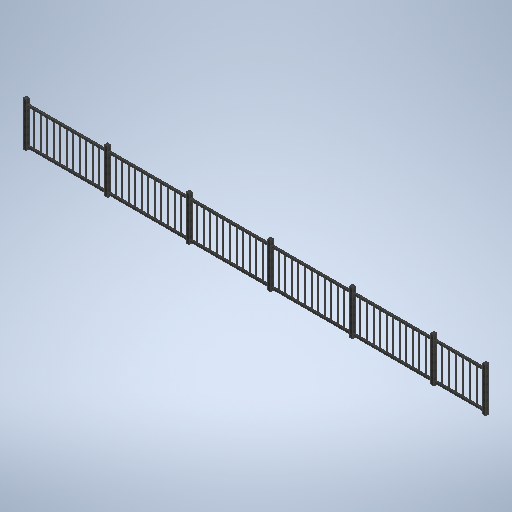
# Autodesk Inventor part: Railing side A
Saved by Autodesk Inventor 2025 (Build 290162000, 162)
## iProperties
Created: 2024-07-15
Part Number: Railing side A
Material: Steel ASTM A36
Document SubType Name: Modeling
Designer: track
Density: 7.85 g/cm^3
Appearance: Plate
Author: track
Autodesk Inventor part; units mm, degrees
ref_plane "YZ Plane" through (0, 0, 0) normal (1, 0, 0) x (0, 1, 0)
ref_plane "XZ Plane" through (0, 0, 0) normal (0, 1, 0) x (-1, 0, 0)
ref_plane "XY Plane" through (0, 0, 0) normal (0, 0, 1) x (1, 0, 0)
sketch "Sketch1" plane through (0, 0, 0) normal (0, 1, 0) x (-1, 0, 0)
  line L0 (-38.1, -38.1) -> (38.1, -38.1)
  line L1 (38.1, -38.1) -> (38.1, 38.1)
  line L2 (38.1, 38.1) -> (-38.1, 38.1)
  line L3 (-38.1, 38.1) -> (-38.1, -38.1)
  line L4 (-38.1, -38.1) -> (38.1, 38.1) construction
  line L5 (38.1, -38.1) -> (-38.1, 38.1) construction
  point P0 (0, 0)
  dimension "d0" = 76.2
  dimension "d1" = 76.2
  constraints: 12 end point, 2 midpoint, 2 parallel, 1 horizontal, 1 perpendicular
  measures "d0" distance of L1.end L2.end
  measures "d1" distance of L0.end L1.end
extrude "Extrusion1" add sketch "Sketch1" along normal blind 1117.6
sketch "Sketch2" plane through (38.1, 0, 38.1) normal (1, 0, 0) x (0, 0, -1)
  line L0 (19.05, 95.25) -> (57.15, 95.25)
  line L1 (57.15, 95.25) -> (57.15, 57.15)
  line L2 (57.15, 57.15) -> (19.05, 57.15)
  line L3 (19.05, 57.15) -> (19.05, 95.25)
  line L4 (19.05, 95.25) -> (57.15, 57.15) construction
  line L5 (57.15, 95.25) -> (19.05, 57.15) construction
  line L6 (19.05, 996.95) -> (57.15, 996.95)
  line L7 (57.15, 996.95) -> (57.15, 958.85)
  line L8 (57.15, 958.85) -> (19.05, 958.85)
  line L9 (19.05, 958.85) -> (19.05, 996.95)
  line L10 (19.05, 996.95) -> (57.15, 958.85) construction
  line L11 (57.15, 996.95) -> (19.05, 958.85) construction
  line L12 (76.2, 329.1929) -> (76.2, 1461.8329)
  line L13 (76.2, 282.1305) -> (76.2, 1152.2607)
  line L14 (76.2, 0) -> (76.2, 1117.6) projected
  line L15 (0, 0) -> (76.2, 0) projected
  point P0 (38.1, 0)
  point P1 (-393.2293, 273.1932)
  point P2 (483.6892, 252.9929)
  point P3 (38.1, 76.2)
  point P4 (38.1, 977.9)
  dimension "d4" = 38.1
  dimension "d5" = 38.1
  dimension "d6" = 38.1
  dimension "d7" = 863.6
  dimension "d8" = 38.1
  dimension "d9" = 38.1
  dimension "d10" = 38.1
  dimension "d12" = 76.2
  constraints: 28 end point, 4 midpoint, 4 parallel, 2 horizontal, 2 perpendicular, 1 collinear, 1 point on line, 1 vertical
  measures "d4" distance of L0.end L1.end
  measures "d5" distance of L0.start L0.end
  measures "d6" distance from line of L12 point (38.1, 76.2)
  measures "d7" distance between parallel lines of L8 L0
  measures "d8" distance of L6.end L7.end
  measures "d9" distance of L6.start L6.end
  measures "d10" distance from line of L13 point (38.1, 977.9)
  measures "d12" distance from line of L15 point (38.1, 76.2)
extrude "Extrusion2" add sketch "Sketch2" along normal blind 1974.85
sketch "Sketch3" plane through (0, 0, 0) normal (0, 1, 0) x (-1, 0, 0)
  line L0 (0, 0) -> (-2051.05, 0)
  line L1 (-38.1, -19.05) -> (-2012.95, -19.05) projected
  line L2 (-2012.95, 38.1) -> (-2089.15, 38.1)
  line L3 (-2089.15, 38.1) -> (-2089.15, -38.1)
  line L4 (-2089.15, -38.1) -> (-2012.95, -38.1)
  line L5 (-2012.95, -38.1) -> (-2012.95, 38.1)
  line L6 (-2012.95, 38.1) -> (-2089.15, -38.1) construction
  line L7 (-2089.15, 38.1) -> (-2012.95, -38.1) construction
  line L8 (-2012.95, -19.05) -> (-2012.95, 19.05) projected
  dimension "d15" = 76.2
  dimension "d16" = 76.2
  constraints: 14 end point, 3 parallel, 2 midpoint, 1 collinear, 1 horizontal, 1 perpendicular
  measures "d15" distance of L3.end L4.end
  measures "d16" distance of L2.end L3.end
extrude "Extrusion3" add sketch "Sketch3" along normal blind 1117.6
sketch "Sketch4" plane through (2089.15, 0, 38.1) normal (1, 0, 0) x (0, 0, -1)
  line L0 (57.15, 996.95) -> (57.15, 958.85) projected
  line L1 (57.15, 958.85) -> (57.15, 996.95) projected
  line L2 (19.05, 996.95) -> (57.15, 996.95) projected
  line L3 (57.15, 996.95) -> (19.05, 996.95) projected
  line L4 (19.05, 958.85) -> (19.05, 996.95) projected
  line L5 (19.05, 996.95) -> (19.05, 958.85) projected
  line L6 (57.15, 958.85) -> (19.05, 958.85) projected
  line L7 (19.05, 958.85) -> (57.15, 958.85) projected
  line L8 (57.15, 57.15) -> (19.05, 57.15) projected
  line L9 (19.05, 57.15) -> (57.15, 57.15) projected
  line L10 (19.05, 57.15) -> (19.05, 95.25) projected
  line L11 (19.05, 95.25) -> (19.05, 57.15) projected
  line L12 (19.05, 95.25) -> (57.15, 95.25) projected
  line L13 (57.15, 95.25) -> (19.05, 95.25) projected
  line L14 (57.15, 95.25) -> (57.15, 57.15) projected
  line L15 (57.15, 57.15) -> (57.15, 95.25) projected
  line L16 (19.05, 95.25) -> (57.15, 95.25)
  line L17 (57.15, 95.25) -> (57.15, 57.15)
  line L18 (57.15, 57.15) -> (19.05, 57.15)
  line L19 (19.05, 57.15) -> (19.05, 95.25)
  line L20 (19.05, 996.95) -> (57.15, 996.95)
  line L21 (57.15, 996.95) -> (57.15, 958.85)
  line L22 (57.15, 958.85) -> (19.05, 958.85)
  line L23 (19.05, 958.85) -> (19.05, 996.95)
  point P0 (38.1, 0)
  point P1 (19.05, 958.85)
  point P2 (19.05, 996.95)
  point P3 (19.05, 95.25)
  point P4 (19.05, 57.15)
  constraints: 16 end point, 4 parallel, 2 horizontal, 2 perpendicular
extrude "Extrusion4" add sketch "Sketch4" along normal blind 1984.375
sketch "Sketch5" plane through (0, 0, 0) normal (0, 1, 0) x (-1, 0, 0)
  line L0 (-4073.525, -19.05) -> (-4073.525, 19.05) projected
  line L1 (-4073.525, 0) -> (-4111.625, 0)
  line L2 (-4149.725, -38.1) -> (-4073.525, -38.1)
  line L3 (-4073.525, -38.1) -> (-4073.525, 38.1)
  line L4 (-4073.525, 38.1) -> (-4149.725, 38.1)
  line L5 (-4149.725, 38.1) -> (-4149.725, -38.1)
  line L6 (-4149.725, -38.1) -> (-4073.525, 38.1) construction
  line L7 (-4073.525, -38.1) -> (-4149.725, 38.1) construction
  line L8 (-4073.525, -19.05) -> (-4073.525, 19.05) projected
  point P0 (0, 0)
  dimension "d21" = 76.2
  dimension "d22" = 76.2
  constraints: 14 end point, 3 midpoint, 2 horizontal, 2 parallel, 1 collinear, 1 perpendicular
  measures "d21" distance of L2.start L2.end
  measures "d22" distance of L4.end L2.start
extrude "Extrusion5" add sketch "Sketch5" along normal blind 1117.6
sketch "Sketch6" plane through (4149.725, 0, 38.1) normal (1, 0, 0) x (0, 0, -1)
  line L0 (19.05, 95.25) -> (57.15, 95.25) projected
  line L1 (57.15, 95.25) -> (19.05, 95.25) projected
  line L2 (19.05, 57.15) -> (19.05, 95.25) projected
  line L3 (19.05, 95.25) -> (19.05, 57.15) projected
  line L4 (57.15, 95.25) -> (57.15, 57.15) projected
  line L5 (57.15, 57.15) -> (57.15, 95.25) projected
  line L6 (57.15, 57.15) -> (19.05, 57.15) projected
  line L7 (19.05, 57.15) -> (57.15, 57.15) projected
  line L8 (57.15, 996.95) -> (57.15, 958.85) projected
  line L9 (57.15, 958.85) -> (57.15, 996.95) projected
  line L10 (57.15, 958.85) -> (19.05, 958.85) projected
  line L11 (19.05, 958.85) -> (57.15, 958.85) projected
  line L12 (19.05, 996.95) -> (57.15, 996.95) projected
  line L13 (57.15, 996.95) -> (19.05, 996.95) projected
  line L14 (19.05, 958.85) -> (19.05, 996.95) projected
  line L15 (19.05, 996.95) -> (19.05, 958.85) projected
  point P0 (38.1, 0)
extrude "Extrusion6" add sketch "Sketch6" along normal blind 1984.375
sketch "Sketch7" plane through (0, 0, 0) normal (0, 1, 0) x (-1, 0, 0)
  line L0 (-6134.1, 19.05) -> (-6134.1, -19.05) projected
  line L1 (-6134.1, 0) -> (-6172.2, 0)
  line L2 (-6134.1, 38.1) -> (-6210.3, 38.1)
  line L3 (-6210.3, 38.1) -> (-6210.3, -38.1)
  line L4 (-6210.3, -38.1) -> (-6134.1, -38.1)
  line L5 (-6134.1, -38.1) -> (-6134.1, 38.1)
  line L6 (-6134.1, 38.1) -> (-6210.3, -38.1) construction
  line L7 (-6210.3, 38.1) -> (-6134.1, -38.1) construction
  line L8 (-6134.1, -19.05) -> (-6134.1, 19.05) projected
  point P0 (0, 0)
  dimension "d27" = 76.2
  dimension "d28" = 76.2
  constraints: 14 end point, 3 midpoint, 2 horizontal, 2 parallel, 1 collinear, 1 perpendicular
  measures "d27" distance of L4.end L2.start
  measures "d28" distance of L3.end L4.end
extrude "Extrusion7" add sketch "Sketch7" along normal blind 1117.6
sketch "Sketch8" plane through (6210.3, 0, 38.1) normal (1, 0, 0) x (0, 0, -1)
  line L0 (19.05, 958.85) -> (19.05, 996.95) projected
  line L1 (19.05, 996.95) -> (19.05, 958.85) projected
  line L2 (19.05, 996.95) -> (57.15, 996.95) projected
  line L3 (57.15, 996.95) -> (19.05, 996.95) projected
  line L4 (57.15, 996.95) -> (57.15, 958.85) projected
  line L5 (57.15, 958.85) -> (57.15, 996.95) projected
  line L6 (57.15, 958.85) -> (19.05, 958.85) projected
  line L7 (19.05, 958.85) -> (57.15, 958.85) projected
  line L8 (57.15, 95.25) -> (57.15, 57.15) projected
  line L9 (57.15, 57.15) -> (57.15, 95.25) projected
  line L10 (57.15, 57.15) -> (19.05, 57.15) projected
  line L11 (19.05, 57.15) -> (57.15, 57.15) projected
  line L12 (19.05, 95.25) -> (57.15, 95.25) projected
  line L13 (57.15, 95.25) -> (19.05, 95.25) projected
  line L14 (19.05, 57.15) -> (19.05, 95.25) projected
  line L15 (19.05, 95.25) -> (19.05, 57.15) projected
  point P0 (38.1, 0)
extrude "Extrusion8" add sketch "Sketch8" along normal blind 1984.375
sketch "Sketch9" plane through (0, 0, 0) normal (0, 1, 0) x (-1, 0, 0)
  line L0 (-8194.675, 19.05) -> (-8194.675, -19.05) projected
  line L1 (-8194.675, 0) -> (-8232.775, 0)
  line L2 (-8194.675, 38.1) -> (-8270.875, 38.1)
  line L3 (-8270.875, 38.1) -> (-8270.875, -38.1)
  line L4 (-8270.875, -38.1) -> (-8194.675, -38.1)
  line L5 (-8194.675, -38.1) -> (-8194.675, 38.1)
  line L6 (-8194.675, 38.1) -> (-8270.875, -38.1) construction
  line L7 (-8270.875, 38.1) -> (-8194.675, -38.1) construction
  line L8 (-8194.675, -19.05) -> (-8194.675, 19.05) projected
  point P0 (0, 0)
  dimension "d33" = 76.2
  dimension "d34" = 76.2
  constraints: 14 end point, 3 midpoint, 2 horizontal, 2 parallel, 1 collinear, 1 perpendicular
  measures "d33" distance of L3.end L4.end
  measures "d34" distance of L4.end L2.start
extrude "Extrusion9" add sketch "Sketch9" along normal blind 1117.6
sketch "Sketch10" plane through (8270.875, 0, 38.1) normal (1, 0, 0) x (0, 0, -1)
  line L0 (19.05, 57.15) -> (19.05, 95.25) projected
  line L1 (19.05, 95.25) -> (19.05, 57.15) projected
  line L2 (19.05, 95.25) -> (57.15, 95.25) projected
  line L3 (57.15, 95.25) -> (19.05, 95.25) projected
  line L4 (57.15, 95.25) -> (57.15, 57.15) projected
  line L5 (57.15, 57.15) -> (57.15, 95.25) projected
  line L6 (57.15, 57.15) -> (19.05, 57.15) projected
  line L7 (19.05, 57.15) -> (57.15, 57.15) projected
  line L8 (57.15, 958.85) -> (19.05, 958.85) projected
  line L9 (19.05, 958.85) -> (57.15, 958.85) projected
  line L10 (57.15, 996.95) -> (57.15, 958.85) projected
  line L11 (57.15, 958.85) -> (57.15, 996.95) projected
  line L12 (19.05, 996.95) -> (57.15, 996.95) projected
  line L13 (57.15, 996.95) -> (19.05, 996.95) projected
  line L14 (19.05, 958.85) -> (19.05, 996.95) projected
  line L15 (19.05, 996.95) -> (19.05, 958.85) projected
  point P0 (38.1, 0)
extrude "Extrusion10" add sketch "Sketch10" along normal blind 1981.2
sketch "Sketch11" plane through (0, 0, 0) normal (0, 1, 0) x (-1, 0, 0)
  line L0 (-10252.075, 19.05) -> (-10252.075, -19.05) projected
  line L1 (-10252.075, 0) -> (-10290.175, 0)
  line L2 (-10328.275, 38.1) -> (-10252.075, 38.1)
  line L3 (-10252.075, 38.1) -> (-10252.075, -38.1)
  line L4 (-10252.075, -38.1) -> (-10328.275, -38.1)
  line L5 (-10328.275, -38.1) -> (-10328.275, 38.1)
  line L6 (-10328.275, 38.1) -> (-10252.075, -38.1) construction
  line L7 (-10252.075, 38.1) -> (-10328.275, -38.1) construction
  line L8 (-10252.075, -19.05) -> (-10252.075, 19.05) projected
  point P0 (0, 0)
  dimension "d39" = 76.2
  dimension "d40" = 76.2
  constraints: 14 end point, 3 midpoint, 2 horizontal, 2 parallel, 1 collinear, 1 perpendicular
  measures "d39" distance of L4.end L2.start
  measures "d40" distance of L3.end L4.end
extrude "Extrusion11" add sketch "Sketch11" along normal blind 1117.6
sketch "Sketch12" plane through (10328.275, 0, 38.1) normal (1, 0, 0) x (0, 0, -1)
  line L0 (19.05, 57.15) -> (19.05, 95.25) projected
  line L1 (19.05, 95.25) -> (19.05, 57.15) projected
  line L2 (19.05, 95.25) -> (57.15, 95.25) projected
  line L3 (57.15, 95.25) -> (19.05, 95.25) projected
  line L4 (57.15, 95.25) -> (57.15, 57.15) projected
  line L5 (57.15, 57.15) -> (57.15, 95.25) projected
  line L6 (57.15, 57.15) -> (19.05, 57.15) projected
  line L7 (19.05, 57.15) -> (57.15, 57.15) projected
  line L8 (57.15, 958.85) -> (19.05, 958.85) projected
  line L9 (19.05, 958.85) -> (57.15, 958.85) projected
  line L10 (57.15, 996.95) -> (57.15, 958.85) projected
  line L11 (57.15, 958.85) -> (57.15, 996.95) projected
  line L12 (19.05, 996.95) -> (57.15, 996.95) projected
  line L13 (57.15, 996.95) -> (19.05, 996.95) projected
  line L14 (19.05, 958.85) -> (19.05, 996.95) projected
  line L15 (19.05, 996.95) -> (19.05, 958.85) projected
  point P0 (38.1, 0)
  point P1 (76.2, 0)
extrude "Extrusion12" add sketch "Sketch12" along normal blind 1231.9
sketch "Sketch13" plane through (0, 0, 0) normal (0, 1, 0) x (-1, 0, 0)
  line L0 (-11560.175, 19.05) -> (-11560.175, -19.05) projected
  line L1 (-11560.175, 0) -> (-11598.275, 0)
  line L2 (-11560.175, 38.1) -> (-11636.375, 38.1)
  line L3 (-11636.375, 38.1) -> (-11636.375, -38.1)
  line L4 (-11636.375, -38.1) -> (-11560.175, -38.1)
  line L5 (-11560.175, -38.1) -> (-11560.175, 38.1)
  line L6 (-11560.175, 38.1) -> (-11636.375, -38.1) construction
  line L7 (-11636.375, 38.1) -> (-11560.175, -38.1) construction
  line L8 (-11560.175, -19.05) -> (-11560.175, 19.05) projected
  point P0 (0, 0)
  dimension "d45" = 76.2
  dimension "d46" = 76.2
  constraints: 14 end point, 3 midpoint, 2 horizontal, 2 parallel, 1 collinear, 1 perpendicular
  measures "d45" distance of L3.end L4.end
  measures "d46" distance of L2.end L3.end
extrude "Extrusion13" add sketch "Sketch13" along normal blind 1117.6
sketch "Sketch14" plane through (38.1, 95.25, 19.05) normal (0, 1, 0) x (1, 0, 0)
  line L0 (0, 0) -> (0, 38.1) projected
  line L1 (0, 19.05) -> (11598.275, 19.05) construction
  line L2 (11598.275, -19.05) -> (11598.275, 57.15) projected
  line L3 (158.2208, 12.7) -> (170.9208, 12.7)
  line L4 (170.9208, 12.7) -> (170.9208, 25.4)
  line L5 (170.9208, 25.4) -> (158.2208, 25.4)
  line L6 (158.2208, 25.4) -> (158.2208, 12.7)
  line L7 (158.2208, 12.7) -> (170.9208, 25.4) construction
  line L8 (170.9208, 12.7) -> (158.2208, 25.4) construction
  line L9 (322.7917, 12.7) -> (335.4917, 12.7)
  line L10 (335.4917, 12.7) -> (335.4917, 25.4)
  line L11 (335.4917, 25.4) -> (322.7917, 25.4)
  line L12 (322.7917, 25.4) -> (322.7917, 12.7)
  line L13 (487.3625, 12.7) -> (500.0625, 12.7)
  line L14 (500.0625, 12.7) -> (500.0625, 25.4)
  line L15 (500.0625, 25.4) -> (487.3625, 25.4)
  line L16 (487.3625, 25.4) -> (487.3625, 12.7)
  line L17 (651.9333, 12.7) -> (664.6333, 12.7)
  line L18 (664.6333, 12.7) -> (664.6333, 25.4)
  line L19 (664.6333, 25.4) -> (651.9333, 25.4)
  line L20 (651.9333, 25.4) -> (651.9333, 12.7)
  line L21 (816.5042, 12.7) -> (829.2042, 12.7)
  line L22 (829.2042, 12.7) -> (829.2042, 25.4)
  line L23 (829.2042, 25.4) -> (816.5042, 25.4)
  line L24 (816.5042, 25.4) -> (816.5042, 12.7)
  line L25 (981.075, 12.7) -> (993.775, 12.7)
  line L26 (993.775, 12.7) -> (993.775, 25.4)
  line L27 (993.775, 25.4) -> (981.075, 25.4)
  line L28 (981.075, 25.4) -> (981.075, 12.7)
  line L29 (1145.6458, 12.7) -> (1158.3458, 12.7)
  line L30 (1158.3458, 12.7) -> (1158.3458, 25.4)
  line L31 (1158.3458, 25.4) -> (1145.6458, 25.4)
  line L32 (1145.6458, 25.4) -> (1145.6458, 12.7)
  line L33 (1310.2167, 12.7) -> (1322.9167, 12.7)
  line L34 (1322.9167, 12.7) -> (1322.9167, 25.4)
  line L35 (1322.9167, 25.4) -> (1310.2167, 25.4)
  line L36 (1310.2167, 25.4) -> (1310.2167, 12.7)
  line L37 (1474.7875, 12.7) -> (1487.4875, 12.7)
  line L38 (1487.4875, 12.7) -> (1487.4875, 25.4)
  line L39 (1487.4875, 25.4) -> (1474.7875, 25.4)
  line L40 (1474.7875, 25.4) -> (1474.7875, 12.7)
  line L41 (1639.3583, 12.7) -> (1652.0583, 12.7)
  line L42 (1652.0583, 12.7) -> (1652.0583, 25.4)
  line L43 (1652.0583, 25.4) -> (1639.3583, 25.4)
  line L44 (1639.3583, 25.4) -> (1639.3583, 12.7)
  line L45 (1803.9292, 12.7) -> (1816.6292, 12.7)
  line L46 (1816.6292, 12.7) -> (1816.6292, 25.4)
  line L47 (1816.6292, 25.4) -> (1803.9292, 25.4)
  line L48 (1803.9292, 25.4) -> (1803.9292, 12.7)
  line L49 (2210.0646, 12.7) -> (2222.7646, 12.7)
  line L50 (2222.7646, 12.7) -> (2222.7646, 25.4)
  line L51 (2222.7646, 25.4) -> (2210.0646, 25.4)
  line L52 (2210.0646, 25.4) -> (2210.0646, 12.7)
  line L53 (2210.0646, 12.7) -> (2222.7646, 25.4) construction
  line L54 (2222.7646, 12.7) -> (2210.0646, 25.4) construction
  line L55 (2051.05, 0) -> (2051.05, 38.1) projected
  line L56 (2388.1292, 25.4) -> (2375.4292, 25.4)
  line L57 (2375.4292, 25.4) -> (2375.4292, 12.7)
  line L58 (2388.1292, 12.7) -> (2388.1292, 25.4)
  line L59 (2375.4292, 12.7) -> (2388.1292, 12.7)
  line L60 (2553.4938, 25.4) -> (2540.7938, 25.4)
  line L61 (2540.7938, 25.4) -> (2540.7938, 12.7)
  line L62 (2553.4938, 12.7) -> (2553.4938, 25.4)
  line L63 (2540.7938, 12.7) -> (2553.4938, 12.7)
  line L64 (2718.8583, 25.4) -> (2706.1583, 25.4)
  line L65 (2706.1583, 25.4) -> (2706.1583, 12.7)
  line L66 (2718.8583, 12.7) -> (2718.8583, 25.4)
  line L67 (2706.1583, 12.7) -> (2718.8583, 12.7)
  line L68 (2884.2229, 25.4) -> (2871.5229, 25.4)
  line L69 (2871.5229, 25.4) -> (2871.5229, 12.7)
  line L70 (2884.2229, 12.7) -> (2884.2229, 25.4)
  line L71 (2871.5229, 12.7) -> (2884.2229, 12.7)
  line L72 (3049.5875, 25.4) -> (3036.8875, 25.4)
  line L73 (3036.8875, 25.4) -> (3036.8875, 12.7)
  line L74 (3049.5875, 12.7) -> (3049.5875, 25.4)
  line L75 (3036.8875, 12.7) -> (3049.5875, 12.7)
  line L76 (3214.9521, 25.4) -> (3202.2521, 25.4)
  line L77 (3202.2521, 25.4) -> (3202.2521, 12.7)
  line L78 (3214.9521, 12.7) -> (3214.9521, 25.4)
  line L79 (3202.2521, 12.7) -> (3214.9521, 12.7)
  line L80 (3380.3167, 25.4) -> (3367.6167, 25.4)
  line L81 (3367.6167, 25.4) -> (3367.6167, 12.7)
  line L82 (3380.3167, 12.7) -> (3380.3167, 25.4)
  line L83 (3367.6167, 12.7) -> (3380.3167, 12.7)
  line L84 (3545.6813, 25.4) -> (3532.9813, 25.4)
  line L85 (3532.9813, 25.4) -> (3532.9813, 12.7)
  line L86 (3545.6813, 12.7) -> (3545.6813, 25.4)
  line L87 (3532.9813, 12.7) -> (3545.6813, 12.7)
  line L88 (3711.0458, 25.4) -> (3698.3458, 25.4)
  line L89 (3698.3458, 25.4) -> (3698.3458, 12.7)
  line L90 (3711.0458, 12.7) -> (3711.0458, 25.4)
  line L91 (3698.3458, 12.7) -> (3711.0458, 12.7)
  line L92 (3876.4104, 25.4) -> (3863.7104, 25.4)
  line L93 (3863.7104, 25.4) -> (3863.7104, 12.7)
  line L94 (3876.4104, 12.7) -> (3876.4104, 25.4)
  line L95 (3863.7104, 12.7) -> (3876.4104, 12.7)
  line L96 (4270.6396, 12.7) -> (4283.3396, 12.7)
  line L97 (4283.3396, 12.7) -> (4283.3396, 25.4)
  line L98 (4283.3396, 25.4) -> (4270.6396, 25.4)
  line L99 (4270.6396, 25.4) -> (4270.6396, 12.7)
  line L100 (4270.6396, 12.7) -> (4283.3396, 25.4) construction
  line L101 (4283.3396, 12.7) -> (4270.6396, 25.4) construction
  line L102 (4111.625, 0) -> (4111.625, 38.1) projected
  line L103 (4448.7042, 12.7) -> (4448.7042, 25.4)
  line L104 (4448.7042, 25.4) -> (4436.0042, 25.4)
  line L105 (4436.0042, 25.4) -> (4436.0042, 12.7)
  line L106 (4436.0042, 12.7) -> (4448.7042, 12.7)
  line L107 (4614.0688, 12.7) -> (4614.0688, 25.4)
  line L108 (4614.0688, 25.4) -> (4601.3688, 25.4)
  line L109 (4601.3688, 25.4) -> (4601.3688, 12.7)
  line L110 (4601.3688, 12.7) -> (4614.0688, 12.7)
  line L111 (4779.4333, 12.7) -> (4779.4333, 25.4)
  line L112 (4779.4333, 25.4) -> (4766.7333, 25.4)
  line L113 (4766.7333, 25.4) -> (4766.7333, 12.7)
  line L114 (4766.7333, 12.7) -> (4779.4333, 12.7)
  line L115 (4944.7979, 12.7) -> (4944.7979, 25.4)
  line L116 (4944.7979, 25.4) -> (4932.0979, 25.4)
  line L117 (4932.0979, 25.4) -> (4932.0979, 12.7)
  line L118 (4932.0979, 12.7) -> (4944.7979, 12.7)
  line L119 (5110.1625, 12.7) -> (5110.1625, 25.4)
  line L120 (5110.1625, 25.4) -> (5097.4625, 25.4)
  line L121 (5097.4625, 25.4) -> (5097.4625, 12.7)
  line L122 (5097.4625, 12.7) -> (5110.1625, 12.7)
  line L123 (5275.5271, 12.7) -> (5275.5271, 25.4)
  line L124 (5275.5271, 25.4) -> (5262.8271, 25.4)
  line L125 (5262.8271, 25.4) -> (5262.8271, 12.7)
  line L126 (5262.8271, 12.7) -> (5275.5271, 12.7)
  line L127 (5440.8917, 12.7) -> (5440.8917, 25.4)
  line L128 (5440.8917, 25.4) -> (5428.1917, 25.4)
  line L129 (5428.1917, 25.4) -> (5428.1917, 12.7)
  line L130 (5428.1917, 12.7) -> (5440.8917, 12.7)
  line L131 (5606.2563, 12.7) -> (5606.2563, 25.4)
  line L132 (5606.2563, 25.4) -> (5593.5563, 25.4)
  line L133 (5593.5563, 25.4) -> (5593.5563, 12.7)
  line L134 (5593.5563, 12.7) -> (5606.2563, 12.7)
  line L135 (5771.6208, 12.7) -> (5771.6208, 25.4)
  line L136 (5771.6208, 25.4) -> (5758.9208, 25.4)
  line L137 (5758.9208, 25.4) -> (5758.9208, 12.7)
  line L138 (5758.9208, 12.7) -> (5771.6208, 12.7)
  line L139 (5936.9854, 12.7) -> (5936.9854, 25.4)
  line L140 (5936.9854, 25.4) -> (5924.2854, 25.4)
  line L141 (5924.2854, 25.4) -> (5924.2854, 12.7)
  line L142 (5924.2854, 12.7) -> (5936.9854, 12.7)
  line L143 (6331.2146, 12.7) -> (6343.9146, 12.7)
  line L144 (6343.9146, 12.7) -> (6343.9146, 25.4)
  line L145 (6343.9146, 25.4) -> (6331.2146, 25.4)
  line L146 (6331.2146, 25.4) -> (6331.2146, 12.7)
  line L147 (6331.2146, 12.7) -> (6343.9146, 25.4) construction
  line L148 (6343.9146, 12.7) -> (6331.2146, 25.4) construction
  line L149 (6172.2, 0) -> (6172.2, 38.1) projected
  line L150 (6509.2792, 25.4) -> (6496.5792, 25.4)
  line L151 (6509.2792, 12.7) -> (6509.2792, 25.4)
  line L152 (6496.5792, 25.4) -> (6496.5792, 12.7)
  line L153 (6496.5792, 12.7) -> (6509.2792, 12.7)
  line L154 (6674.6438, 25.4) -> (6661.9438, 25.4)
  line L155 (6674.6438, 12.7) -> (6674.6438, 25.4)
  line L156 (6661.9438, 25.4) -> (6661.9438, 12.7)
  line L157 (6661.9438, 12.7) -> (6674.6438, 12.7)
  line L158 (6840.0083, 25.4) -> (6827.3083, 25.4)
  line L159 (6840.0083, 12.7) -> (6840.0083, 25.4)
  line L160 (6827.3083, 25.4) -> (6827.3083, 12.7)
  line L161 (6827.3083, 12.7) -> (6840.0083, 12.7)
  line L162 (7005.3729, 25.4) -> (6992.6729, 25.4)
  line L163 (7005.3729, 12.7) -> (7005.3729, 25.4)
  line L164 (6992.6729, 25.4) -> (6992.6729, 12.7)
  line L165 (6992.6729, 12.7) -> (7005.3729, 12.7)
  line L166 (7170.7375, 25.4) -> (7158.0375, 25.4)
  line L167 (7170.7375, 12.7) -> (7170.7375, 25.4)
  line L168 (7158.0375, 25.4) -> (7158.0375, 12.7)
  line L169 (7158.0375, 12.7) -> (7170.7375, 12.7)
  line L170 (7336.1021, 25.4) -> (7323.4021, 25.4)
  line L171 (7336.1021, 12.7) -> (7336.1021, 25.4)
  line L172 (7323.4021, 25.4) -> (7323.4021, 12.7)
  line L173 (7323.4021, 12.7) -> (7336.1021, 12.7)
  line L174 (7501.4667, 25.4) -> (7488.7667, 25.4)
  line L175 (7501.4667, 12.7) -> (7501.4667, 25.4)
  line L176 (7488.7667, 25.4) -> (7488.7667, 12.7)
  line L177 (7488.7667, 12.7) -> (7501.4667, 12.7)
  line L178 (7666.8313, 25.4) -> (7654.1313, 25.4)
  line L179 (7666.8313, 12.7) -> (7666.8313, 25.4)
  line L180 (7654.1313, 25.4) -> (7654.1313, 12.7)
  line L181 (7654.1313, 12.7) -> (7666.8313, 12.7)
  line L182 (7832.1958, 25.4) -> (7819.4958, 25.4)
  line L183 (7832.1958, 12.7) -> (7832.1958, 25.4)
  line L184 (7819.4958, 25.4) -> (7819.4958, 12.7)
  line L185 (7819.4958, 12.7) -> (7832.1958, 12.7)
  line L186 (7997.5604, 25.4) -> (7984.8604, 25.4)
  line L187 (7997.5604, 12.7) -> (7997.5604, 25.4)
  line L188 (7984.8604, 25.4) -> (7984.8604, 12.7)
  line L189 (7984.8604, 12.7) -> (7997.5604, 12.7)
  line L190 (8391.525, 12.7) -> (8404.225, 12.7)
  line L191 (8404.225, 12.7) -> (8404.225, 25.4)
  line L192 (8404.225, 25.4) -> (8391.525, 25.4)
  line L193 (8391.525, 25.4) -> (8391.525, 12.7)
  line L194 (8391.525, 12.7) -> (8404.225, 25.4) construction
  line L195 (8404.225, 12.7) -> (8391.525, 25.4) construction
  line L196 (8232.775, 0) -> (8232.775, 38.1) projected
  line L197 (8569.325, 12.7) -> (8569.325, 25.4)
  line L198 (8569.325, 25.4) -> (8556.625, 25.4)
  line L199 (8556.625, 25.4) -> (8556.625, 12.7)
  line L200 (8556.625, 12.7) -> (8569.325, 12.7)
  line L201 (8734.425, 12.7) -> (8734.425, 25.4)
  line L202 (8734.425, 25.4) -> (8721.725, 25.4)
  line L203 (8721.725, 25.4) -> (8721.725, 12.7)
  line L204 (8721.725, 12.7) -> (8734.425, 12.7)
  line L205 (8899.525, 12.7) -> (8899.525, 25.4)
  line L206 (8899.525, 25.4) -> (8886.825, 25.4)
  line L207 (8886.825, 25.4) -> (8886.825, 12.7)
  line L208 (8886.825, 12.7) -> (8899.525, 12.7)
  line L209 (9064.625, 12.7) -> (9064.625, 25.4)
  line L210 (9064.625, 25.4) -> (9051.925, 25.4)
  line L211 (9051.925, 25.4) -> (9051.925, 12.7)
  line L212 (9051.925, 12.7) -> (9064.625, 12.7)
  line L213 (9229.725, 12.7) -> (9229.725, 25.4)
  line L214 (9229.725, 25.4) -> (9217.025, 25.4)
  line L215 (9217.025, 25.4) -> (9217.025, 12.7)
  line L216 (9217.025, 12.7) -> (9229.725, 12.7)
  line L217 (9394.825, 12.7) -> (9394.825, 25.4)
  line L218 (9394.825, 25.4) -> (9382.125, 25.4)
  line L219 (9382.125, 25.4) -> (9382.125, 12.7)
  line L220 (9382.125, 12.7) -> (9394.825, 12.7)
  line L221 (9559.925, 12.7) -> (9559.925, 25.4)
  line L222 (9559.925, 25.4) -> (9547.225, 25.4)
  line L223 (9547.225, 25.4) -> (9547.225, 12.7)
  line L224 (9547.225, 12.7) -> (9559.925, 12.7)
  line L225 (9725.025, 12.7) -> (9725.025, 25.4)
  line L226 (9725.025, 25.4) -> (9712.325, 25.4)
  line L227 (9712.325, 25.4) -> (9712.325, 12.7)
  line L228 (9712.325, 12.7) -> (9725.025, 12.7)
  line L229 (9890.125, 12.7) -> (9890.125, 25.4)
  line L230 (9890.125, 25.4) -> (9877.425, 25.4)
  line L231 (9877.425, 25.4) -> (9877.425, 12.7)
  line L232 (9877.425, 12.7) -> (9890.125, 12.7)
  line L233 (10055.225, 12.7) -> (10055.225, 25.4)
  line L234 (10055.225, 25.4) -> (10042.525, 25.4)
  line L235 (10042.525, 25.4) -> (10042.525, 12.7)
  line L236 (10042.525, 12.7) -> (10055.225, 12.7)
  line L237 (10459.8107, 12.7) -> (10472.5107, 12.7)
  line L238 (10472.5107, 12.7) -> (10472.5107, 25.4)
  line L239 (10472.5107, 25.4) -> (10459.8107, 25.4)
  line L240 (10459.8107, 25.4) -> (10459.8107, 12.7)
  line L241 (10459.8107, 12.7) -> (10472.5107, 25.4) construction
  line L242 (10472.5107, 12.7) -> (10459.8107, 25.4) construction
  line L243 (10290.175, 0) -> (10290.175, 38.1) projected
  line L244 (10648.4964, 12.7) -> (10648.4964, 25.4)
  line L245 (10648.4964, 25.4) -> (10635.7964, 25.4)
  line L246 (10635.7964, 25.4) -> (10635.7964, 12.7)
  line L247 (10635.7964, 12.7) -> (10648.4964, 12.7)
  line L248 (10824.4821, 12.7) -> (10824.4821, 25.4)
  line L249 (10824.4821, 25.4) -> (10811.7821, 25.4)
  line L250 (10811.7821, 25.4) -> (10811.7821, 12.7)
  line L251 (10811.7821, 12.7) -> (10824.4821, 12.7)
  line L252 (11000.4679, 12.7) -> (11000.4679, 25.4)
  line L253 (11000.4679, 25.4) -> (10987.7679, 25.4)
  line L254 (10987.7679, 25.4) -> (10987.7679, 12.7)
  line L255 (10987.7679, 12.7) -> (11000.4679, 12.7)
  line L256 (11176.4536, 12.7) -> (11176.4536, 25.4)
  line L257 (11176.4536, 25.4) -> (11163.7536, 25.4)
  line L258 (11163.7536, 25.4) -> (11163.7536, 12.7)
  line L259 (11163.7536, 12.7) -> (11176.4536, 12.7)
  line L260 (11352.4393, 12.7) -> (11352.4393, 25.4)
  line L261 (11352.4393, 25.4) -> (11339.7393, 25.4)
  line L262 (11339.7393, 25.4) -> (11339.7393, 12.7)
  line L263 (11339.7393, 12.7) -> (11352.4393, 12.7)
  point P0 (-38.1, 19.05)
  point P1 (164.5708, 19.05)
  point P2 (2216.4146, 19.05)
  point P3 (4276.9896, 19.05)
  point P4 (6337.5646, 19.05)
  point P5 (8397.875, 19.05)
  point P6 (10466.1607, 19.05)
  dimension "d49" = 12.7
  dimension "d50" = 12.7
  dimension "d51" = 164.5708
  dimension "d54" = 164.5708
  dimension "d59" = 12.7
  dimension "d60" = 12.7
  dimension "d61" = 165.3646
  dimension "d64" = 165.3646
  dimension "d69" = 12.7
  dimension "d70" = 12.7
  dimension "d71" = 165.3646
  dimension "d74" = 165.3646
  dimension "d79" = 12.7
  dimension "d80" = 12.7
  dimension "d81" = 165.3646
  dimension "d84" = 165.3646
  dimension "d89" = 12.7
  dimension "d90" = 12.7
  dimension "d91" = 165.1
  dimension "d94" = 165.1
  dimension "d99" = 12.7
  dimension "d100" = 12.7
  dimension "d101" = 175.9857
  dimension "d104" = 175.9857
  constraints: 514 end point, 14 midpoint, 12 horizontal, 12 parallel, 6 perpendicular, 6 point on line, 440 other
  measures "d49" distance of L4.end L5.end
  measures "d50" distance of L3.end L4.end
  measures "d51" distance from line of L0 point (164.571, 19.05)
  measures "d54" distance of L3.start L9.start
  measures "d59" distance of L50.end L51.end
  measures "d60" distance of L49.end L50.end
  measures "d61" distance from line of L55 point (2216.415, 19.05)
  measures "d64" distance of L50.end L56.start
  measures "d69" distance of L97.end L98.end
  measures "d70" distance of L96.end L97.end
  measures "d71" distance from line of L102 point (4276.99, 19.05)
  measures "d74" distance of L96.end L103.start
  measures "d79" distance of L144.end L145.end
  measures "d80" distance of L143.end L144.end
  measures "d81" distance from line of L149 point (6337.565, 19.05)
  measures "d84" distance of L144.end L150.start
  measures "d89" distance of L191.end L192.end
  measures "d90" distance of L190.end L191.end
  measures "d91" distance from line of L196 point (8397.875, 19.05)
  measures "d94" distance of L190.end L197.start
  measures "d99" distance of L238.end L239.end
  measures "d100" distance of L237.end L238.end
  measures "d101" distance from line of L243 point (10466.161, 19.05)
  measures "d104" distance of L237.end L244.start
extrude "Extrusion14" add sketch "Sketch14" along normal up to surface (863.6 mm away)
body "Solid1"
